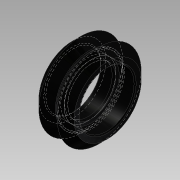
# Autodesk Inventor part: Dual V Wheel
Saved by Autodesk Inventor 2013 SP2 (Build 170200200, 200)
## iProperties
Created: 2013-06-20
Part Number: Dual V Wheel
Material: Acetal Resin, Black
Document SubType Name: Modeling
Designer: Jon Hollander
Density: 1.425 g/cm^3
Mass: 2.60986 g
Surface Area: 18.1288 cm^2
Volume: 1.83148 cm^3
Author: Jon Hollander
Autodesk Inventor part; units mm, degrees
ref_plane "YZ Plane" through (0, 0, 0) normal (1, 0, 0) x (0, 1, 0)
ref_plane "XZ Plane" through (0, 0, 0) normal (0, 1, 0) x (-1, 0, 0)
ref_plane "XY Plane" through (0, 0, 0) normal (0, 0, 1) x (1, 0, 0)
sketch "Sketch1" plane through (0, 0, 0) normal (0, 0, 1) x (1, 0, 0)
  line L0 (0, 0) -> (10, 0)
  line L1 (0, 0) -> (0, 6.945) construction
  line L2 (0, 6.945) -> (0.5, 6.945)
  line L3 (0.5, 6.945) -> (0.5, 7.987)
  line L4 (0.5, 7.987) -> (4.82, 7.987)
  line L5 (5.12, 8.287) -> (5.12, 9.77)
  line L6 (5.12, 9.77) -> (2.695, 12.195)
  line L7 (2.695, 12.195) -> (0.275, 9.775)
  line L8 (0.275, 9.775) -> (0.275, 9.375)
  line L9 (0.275, 9.375) -> (0, 9.375)
  line L10 (4.82, 7.987) -> (5.12, 8.287)
  line L11 (0, 6.945) -> (0, 11.2763) construction
  line L12 (0, 6.945) -> (-0.5, 6.945)
  line L13 (-0.5, 6.945) -> (-0.5, 7.987)
  line L14 (-0.5, 7.987) -> (-4.82, 7.987)
  line L15 (-5.12, 8.287) -> (-5.12, 9.77)
  line L16 (-5.12, 9.77) -> (-2.695, 12.195)
  line L17 (-2.695, 12.195) -> (-0.275, 9.775)
  line L18 (-0.275, 9.775) -> (-0.275, 9.375)
  line L19 (-0.275, 9.375) -> (0, 9.375)
  line L20 (-4.82, 7.987) -> (-5.12, 8.287)
  point P0 (5.12, 7.987)
  point P1 (-5.12, 7.987)
  dimension "d0" = 10
  dimension "d2" = 0.5
  dimension "d3" = 15.974
  dimension "d4" = 13.89
  dimension "d5" = 0.3
  dimension "d6" = 0.3
  dimension "d7" = 19.54
  dimension "d8" = 5.12
  dimension "d12" = 24.39
  dimension "d14" = 18.75
  dimension "d16" = 0.275
  dimension "d17" = 135
  dimension "d18" = 135
  dimension "d19" = 2.695
  constraints: 42 end point, 9 symmetric about line, 5 point on line, 4 parallel, 4 perpendicular, 1 horizontal
  measures "d0" distance of L0.start L0.end
  measures "d2" distance of L1.end L2.end
  measures "d3" diameter of L4 L0
  measures "d4" diameter of L2 L0
  measures "d5" distance of L4.end point (5.12, 7.987)
  measures "d6" distance of L5.start point (5.12, 7.987)
  measures "d7" diameter of L5.end L0
  measures "d8" distance between parallel lines of L1 L5
  measures "d12" diameter of L6.end L0
  measures "d14" diameter of L9 L0
  measures "d16" distance between parallel lines of L11 L8
  measures "d17" angle of L5 L6
  measures "d18" angle of L7 L8
  measures "d19" distance from line of L11 L6.end
revolve "Revolution1" add sketch "Sketch1" angle 360 about axis through (0, 0, 0) along (1, 0, 0)
equation "\"d6\" = d5"
body "Solid1"
